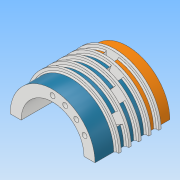
# Autodesk Inventor part: Core
Saved by Autodesk Inventor 2017.3 (Build 213256000, 256)
## iProperties
Created: 2019-05-16
Part Number: Core
Material: ABS Plastic
Document SubType Name: Modeling
Designer: Derek Wider
Density: 1.06 g/cm^3
Appearance: Smooth - White
Author: Derek Wider
Autodesk Inventor part; units mm, degrees
ref_plane "YZ Plane" through (0, 0, 0) normal (1, 0, 0) x (0, 1, 0)
ref_plane "XZ Plane" through (0, 0, 0) normal (0, 1, 0) x (-1, 0, 0)
ref_plane "XY Plane" through (0, 0, 0) normal (0, 0, 1) x (1, 0, 0)
sketch "Sketch1" plane through (0, 0, 0) normal (0, 0, 1) x (1, 0, 0)
  arc A0 (16.002, 0) -> (-16.002, 0) centre (0, 0) ccw
  arc A1 (21.59, 0) -> (-21.59, 0) centre (0, 0) ccw
  line L0 (-16.002, 0) -> (-21.59, 0)
  line L1 (16.002, 0) -> (21.59, 0)
  dimension "d0" = 32.004
  dimension "d1" = 43.18
  constraints: 4 end point, 4 point on circle, 2 centre point, 2 coincident, 2 point on line, 1 horizontal
  measures "d0" diameter of A0
  measures "d1" diameter of A1
extrude "Extrusion1" add sketch "Sketch1" along normal blind 38.1
sketch "Sketch2" plane through (0, 0, 38.1) normal (0, 0, 1) x (1, 0, 0)
  circle A0 centre (16.2778, 9.398) radius 1.27
  line L0 (0, 0) -> (16.2778, 9.398) construction
  line L1 (0, 0) -> (18.796, 0) construction
  circle A1 centre (12.0818, 14.3986) radius 1.27
  circle A2 centre (6.4286, 17.6625) radius 1.27
  circle A3 centre (0, 18.796) radius 1.27
  line L2 (0, 0) -> (12.0818, 14.3986) construction
  line L3 (0, 0) -> (6.4286, 17.6625) construction
  line L4 (0, 0) -> (0, 18.796) construction
  dimension "d4" = 2.54
  dimension "d5" = 18.796
  dimension "d6" = 30
  dimension "d9" = 60
  constraints: 10 end point, 4 centre point, 1 coincident, 1 equal length, 1 horizontal, 7 other
  measures "d4" diameter of A0
  measures "d5" distance of L0.start L0.end
  measures "d6" angle of L1 L0
extrude "Extrusion2" cut sketch "Sketch2" against normal blind 12.7 contours A0
extrude "Extrusion3" cut sketch "Sketch2" against normal blind 19.05 contours A1
extrude "Extrusion4" cut sketch "Sketch2" against normal blind 25.4 contours A2
extrude "Extrusion5" cut sketch "Sketch2" against normal blind 30.48 contours A3
ref_plane "Work Plane4" through (18.6975, 10.795, 0) normal (0.8660254, 0.5, 0) x (-0.5, 0.8660254, 0)
ref_plane "Work Plane3" through (16.2778, 9.398, 38.1) normal (0.8660254, 0.5, 0) x (-0.5, 0.8660254, 0)
sketch "Sketch3" plane through (18.6975, 10.795, 0) normal (0.8660254, 0.5, 0) x (-0.5, 0.8660254, 0)
  line L0 (2.54, 26.67) -> (-2.54, 26.67)
  line L1 (-2.54, 26.67) -> (-2.54, 22.86)
  line L2 (-2.54, 22.86) -> (2.54, 22.86)
  line L3 (2.54, 22.86) -> (2.54, 26.67)
  line L4 (21.59, 38.1) -> (-10.795, 38.1) projected
  point P0 (0, 0)
  point P1 (10.795, 38.1)
  point P2 (0, 22.86)
  dimension "d20" = 11.43
  dimension "d21" = 15.24
  dimension "d22" = 5.08
  constraints: 8 end point, 2 parallel, 1 horizontal, 1 midpoint, 1 perpendicular, 1 vertical alignment
  measures "d20" distance between parallel lines of L4 L0
  measures "d21" distance between parallel lines of L4 L2
  measures "d22" distance between parallel lines of L3 L1
extrude "Extrusion6" cut sketch "Sketch3" against normal blind 4.318
ref_plane "Work Plane7" through (13.8778, 16.5389, 0) normal (0.6427876, 0.7660444, 0) x (-0.7660444, 0.6427876, 0)
ref_plane "Work Plane6" through (12.0818, 14.3986, 38.1) normal (0.6427876, 0.7660444, 0) x (-0.7660444, 0.6427876, 0)
sketch "Sketch4" plane through (13.8778, 16.5389, 0) normal (0.6427876, 0.7660444, 0) x (-0.7660444, 0.6427876, 0)
  line L0 (3.175, 21.59) -> (-3.175, 21.59)
  line L1 (-3.175, 21.59) -> (-3.175, 17.78)
  line L2 (-3.175, 17.78) -> (3.175, 17.78)
  line L3 (3.175, 17.78) -> (3.175, 21.59)
  line L4 (21.59, 38.1) -> (-16.5389, 38.1) projected
  point P0 (0, 0)
  point P1 (0, 17.78)
  point P2 (16.5389, 38.1)
  dimension "d25" = 6.35
  dimension "d26" = 16.51
  dimension "d27" = 20.32
  constraints: 8 end point, 2 parallel, 1 horizontal, 1 midpoint, 1 perpendicular, 1 vertical alignment
  measures "d25" distance of L0.start L0.end
  measures "d26" distance between parallel lines of L4 L0
  measures "d27" distance between parallel lines of L4 L2
extrude "Extrusion7" cut sketch "Sketch4" against normal blind 4.318
ref_plane "Work Plane9" through (7.3842, 20.288, 0) normal (0.3420201, 0.9396926, 0) x (-0.9396926, 0.3420201, 0)
ref_plane "Work Plane8" through (6.4286, 17.6625, 38.1) normal (0.3420201, 0.9396926, 0) x (-0.9396926, 0.3420201, 0)
sketch "Sketch5" plane through (7.3842, 20.288, 0) normal (0.3420201, 0.9396926, 0) x (-0.9396926, 0.3420201, 0)
  line L0 (-3.175, 12.7) -> (3.175, 12.7)
  line L1 (3.175, 12.7) -> (3.175, 16.51)
  line L2 (3.175, 16.51) -> (-3.175, 16.51)
  line L3 (-3.175, 16.51) -> (-3.175, 12.7)
  line L4 (21.59, 38.1) -> (-20.288, 38.1) projected
  point P0 (0, 0)
  point P1 (20.288, 38.1)
  point P2 (0, 12.7)
  dimension "d30" = 6.35
  dimension "d31" = 21.59
  dimension "d32" = 25.4
  constraints: 8 end point, 2 parallel, 1 horizontal, 1 midpoint, 1 perpendicular, 1 vertical alignment
  measures "d30" distance of L1.end L2.end
  measures "d31" distance between parallel lines of L4 L2
  measures "d32" distance between parallel lines of L4 L0
extrude "Extrusion8" cut sketch "Sketch5" against normal blind 4.318
ref_plane "Work Plane11" through (0, 21.59, 0) normal (0, 1, 0) x (-1, 0, 0)
ref_plane "Work Plane10" through (0, 18.796, 38.1) normal (0, 1, 0) x (-1, 0, 0)
sketch "Sketch6" plane through (0, 21.59, 0) normal (0, 1, 0) x (-1, 0, 0)
  line L0 (3.175, 11.43) -> (-3.175, 11.43)
  line L1 (-3.175, 11.43) -> (-3.175, 7.62)
  line L2 (-3.175, 7.62) -> (3.175, 7.62)
  line L3 (3.175, 7.62) -> (3.175, 11.43)
  line L4 (21.59, 0) -> (-21.59, 0) projected
  line L5 (21.59, 38.1) -> (-21.59, 38.1) projected
  point P0 (0, 0)
  point P1 (0, 7.62)
  point P2 (0, 0)
  dimension "d35" = 6.35
  dimension "d36" = 26.67
  dimension "d37" = 30.48
  constraints: 8 end point, 2 midpoint, 2 parallel, 1 horizontal, 1 perpendicular, 1 vertical alignment
  measures "d35" distance of L0.start L0.end
  measures "d36" distance between parallel lines of L5 L0
  measures "d37" distance between parallel lines of L5 L2
sketch "Sketch7" plane through (0, 0, 22.86) normal (0, 0, 1) x (0.8660254, 0.5, 0)
  arc A0 (18.6975, -10.795) -> (-18.6975, 10.795) centre (0, 0) ccw projected
  arc A1 (20.3473, -11.7475) -> (-20.3473, 11.7475) centre (0, 0) ccw
  line L0 (-20.3473, 11.7475) -> (-18.6975, 10.795)
  line L1 (20.3473, -11.7475) -> (18.6975, -10.795)
  dimension "d38" = 1.905
  constraints: 4 end point, 2 point on circle, 1 centre point, 1 collinear
  measures "d38" distance of L0.start L0.end
extrude "Extrusion9" add sketch "Sketch7" against normal blind 1.27
sketch "Sketch8" plane through (0, 0, 17.78) normal (0, 0, 1) x (0.7660444, -0.6427876, 0)
  line L0 (4.9461, 21.0158) -> (3.5206, 17.0991) projected
  line L1 (3.5206, 17.0991) -> (8.2942, 15.3616) projected
  line L2 (9.7198, 19.2783) -> (8.2942, 15.3616) projected
  arc A0 (16.5389, 13.8778) -> (9.7198, 19.2783) centre (0, 0) ccw projected
  line L3 (17.9982, 15.1023) -> (16.5389, 13.8778) projected
  arc A1 (17.9982, 15.1023) -> (-17.9982, -15.1023) centre (0, 0) ccw projected
  line L4 (-16.5389, -13.8778) -> (-17.9982, -15.1023) projected
  arc A2 (4.9461, 21.0158) -> (-16.5389, -13.8778) centre (0, 0) ccw projected
extrude "Extrusion10" add sketch "Sketch8" against normal blind 1.27
sketch "Sketch9" plane through (0, 0, 12.7) normal (0, 0, 1) x (1, 0, 0)
  line L0 (17.2976, 12.9197) -> (13.688, 10.8357) projected
  line L1 (13.688, 10.8357) -> (16.228, 6.4363) projected
  line L2 (19.8376, 8.5203) -> (16.228, 6.4363) projected
  arc A0 (21.59, 0) -> (19.8376, 8.5203) centre (0, 0) ccw projected
  line L3 (23.495, 0) -> (21.59, 0) projected
  arc A1 (23.495, 0) -> (-23.495, 0) centre (0, 0) ccw projected
  line L4 (-21.59, 0) -> (-23.495, 0) projected
  arc A2 (17.2976, 12.9197) -> (-21.59, 0) centre (0, 0) ccw projected
extrude "Extrusion11" add sketch "Sketch9" against normal blind 1.27
extrude "Extrusion12" cut sketch "Sketch6" against normal blind 4.318
sketch "Sketch10" plane through (0, 0, 7.62) normal (0, 0, 1) x (1, 0, 0)
  line L0 (17.2976, 12.9197) -> (13.688, 10.8357) projected
  line L1 (13.688, 10.8357) -> (16.228, 6.4363) projected
  line L2 (19.8376, 8.5203) -> (16.228, 6.4363) projected
  arc A0 (21.59, 0) -> (19.8376, 8.5203) centre (0, 0) ccw projected
  line L3 (23.495, 0) -> (21.59, 0) projected
  arc A1 (23.495, 0) -> (-23.495, 0) centre (0, 0) ccw projected
  line L4 (-21.59, 0) -> (-23.495, 0) projected
  arc A2 (17.2976, 12.9197) -> (-21.59, 0) centre (0, 0) ccw projected
extrude "Extrusion13" add sketch "Sketch10" against normal blind 1.27
sketch "Sketch11" plane through (0, 0, 26.67) normal (0, 0, -1) x (-0.8660254, -0.5, 0)
  arc A0 (18.6975, 10.795) -> (-18.6975, -10.795) centre (0, 0) ccw projected
  line L0 (18.6975, 10.795) -> (20.3473, 11.7475) projected
  arc A1 (20.3473, 11.7475) -> (-20.3473, -11.7475) centre (0, 0) ccw projected
  line L1 (-20.3473, -11.7475) -> (-18.6975, -10.795) projected
extrude "Extrusion14" add sketch "Sketch11" against normal blind 1.27
chamfer "Chamfer1" distance 0.635 angle 45 9 edges at (0, 21.59, 27.94) (-6.8071, 20.4888, 22.86) (-10.5422, 18.8412, 17.78) (-13.6538, 16.7243, 12.7) (-16.3505, 14.0993, 7.62) (16.3505, 14.0993, 7.62) (18.5504, 11.0459, 12.7) (20.1867, 7.6568, 17.78) (21.1474, 4.3493, 22.86)
chamfer "Chamfer2" distance 0.635 angle 45 8 edges at (-6.8071, 20.4888, 26.67) (21.1474, 4.3493, 26.67) (-10.5422, 18.8412, 21.59) (20.1867, 7.6568, 21.59) (-13.6538, 16.7243, 16.51) (18.5504, 11.0459, 16.51) (16.3505, 14.0993, 11.43) (-16.3505, 14.0993, 11.43)
body "Solid1"
